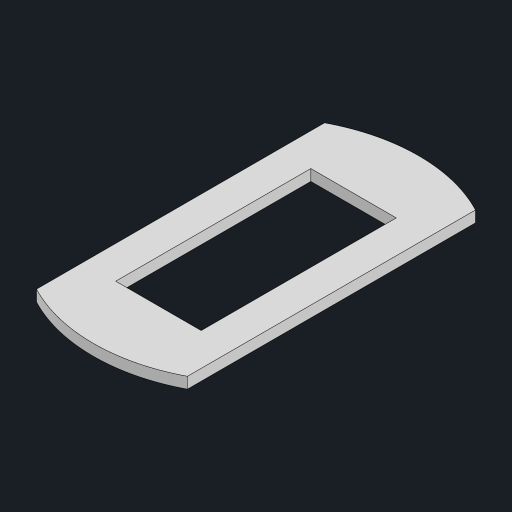
# Autodesk Inventor part: ServoMotor_Holder
Saved by Autodesk Inventor 2023 (Build 270158000, 158)
## iProperties
Created: 2022-07-09
Part Number: ServoMotor_Holder
Material: 一般
Document SubType Name: Modeling
Designer: legot
Density: 1 g/cm^3
Appearance: 既定
Author: legot
Autodesk Inventor part; units mm, degrees
ref_plane "YZ Plane" through (0, 0, 0) normal (1, 0, 0) x (0, 1, 0)
ref_plane "XZ Plane" through (0, 0, 0) normal (0, 1, 0) x (-1, 0, 0)
ref_plane "XY Plane" through (0, 0, 0) normal (0, 0, 1) x (1, 0, 0)
sketch "スケッチ1" plane through (0, 0, 0) normal (0, 1, 0) x (-1, 0, 0)
  circle A0 centre (0, 0) radius 17.5
  line L0 (8.124, 15.5) -> (8.124, -15.5)
  line L1 (-8.124, 15.5) -> (-8.124, -15.5)
  line L2 (4.6, 10.5) -> (-4.6, 10.5)
  line L3 (-4.6, 10.5) -> (-4.6, -10.5)
  line L4 (-4.6, -10.5) -> (4.6, -10.5)
  line L5 (4.6, -10.5) -> (4.6, 10.5)
  point P0 (4.6, 0)
  point P1 (0, 10.5)
  dimension "d0" = 35
  dimension "d1" = 31
  dimension "d2" = 9.2
  dimension "d3" = 21
  constraints: 12 end point, 4 parallel, 4 point on circle, 2 midpoint, 1 centre point, 1 coincident, 1 horizontal, 1 horizontal alignment, 1 perpendicular, 1 vertical, 1 vertical alignment
  measures "d0" diameter of A0
  measures "d1" distance of L0.start L0.end
  measures "d2" distance of L2.start L2.end
  measures "d3" distance of L4.end L2.start
extrude "押し出し1" add sketch "スケッチ1" along normal blind 1.2 contours L0 A0 L1
